Autodesk Inventor part; units mm, degrees
(part 2 of 2)
  dimension "d127" = 22.5
  dimension "d128" = 22.5
  constraints: 820 end point, 471 point on circle, 283 centre point, 40 horizontal, 34 vertical, 31 perpendicular, 9 point on line, 5 equal length, 4 collinear, 2 parallel, 2 tangent
  measures "d65" diameter of A126
  measures "d66" diameter of A127
  measures "d67" distance of L156.start L156.end
  measures "d68" radius of A128
  measures "d69" radius of A129
  measures "d70" distance of L157.start L157.end
  measures "d71" radius of A130
  measures "d72" radius of A131
  measures "d73" distance of L330.end L174.start
  measures "d74" radius of A132
  measures "d75" distance of L4.end L173.start
  measures "d76" radius of A133
  measures "d77" distance of L329.start L171.start
  measures "d78" radius of A134
  measures "d79" distance of L3.start L172.start
  measures "d80" radius of A135
  measures "d81" distance of L166.start L158.end
  measures "d82" distance of L163.start L159.end
  measures "d83" diameter of A136
  measures "d84" diameter of A137
  measures "d85" radius of A138
  measures "d86" radius of A139
  measures "d87" diameter of A141
  measures "d88" distance of L68.end L162.end
  measures "d89" distance of L162.end L164.start
  measures "d90" radius of A142
  measures "d91" distance of L163.end L164.end
  measures "d92" radius of A143
  measures "d93" distance of L64.start L165.end
  measures "d94" distance of L166.end L167.end
  measures "d95" radius of A144
  measures "d96" distance of L165.end L167.start
  measures "d97" radius of A145
  measures "d98" diameter of A146
  measures "d99" diameter of A147
  measures "d100" distance of L168.start L168.end
  measures "d101" distance of L168.end A148.start
  measures "d102" radius of A148
  measures "d103" distance of L169.start L169.end
  measures "d104" distance of L169.end L170.start
  measures "d105" radius of A149
  measures "d106" distance of L170.start L170.end
  measures "d107" radius of A150
  measures "d108" diameter of A151
  measures "d109" diameter of A152
  measures "d110" distance of L171.start L171.end
  measures "d111" distance of L172.start L172.end
  measures "d112" radius of A153
  measures "d113" distance of L173.start L173.end
  measures "d114" distance of L174.start L174.end
  measures "d115" radius of A154
  measures "d116" distance of L8.end L176.end
  measures "d117" distance of L7.start L177.end
  measures "d118" distance of L176.end L180.start
  measures "d119" distance of L177.end L180.end
  measures "d120" diameter of A155
  measures "d121" diameter of A156
  measures "d122" diameter of A157
  measures "d123" diameter of A158
  measures "d124" diameter of A159
  measures "d125" diameter of A160
  measures "d126" diameter of A161
  measures "d127" distance of L188.start L190.end
  measures "d128" distance of L189.start L189.end
extrude "Extrusion2" add sketch "Sketch2" along normal blind 1.5
body "Solid2"
